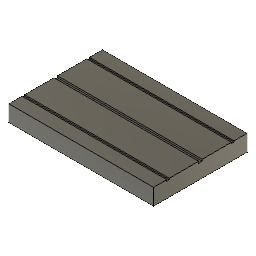
64 Halfsize Breadboard (Autodesk Fusion 360 design; units mm, degrees)
Autodesk Fusion 360 part; units mm, degrees
sketch "Sketch1" plane through (0, 0, 0) normal (0, 0, 1) x (1, 0, 0)
  line L0 (0, 0) -> (85, 0)
  line L1 (85, 0) -> (85, 55)
  line L2 (85, 55) -> (0, 55)
  line L3 (0, 55) -> (0, 0)
  dimension "d1" = 85
  dimension "d2" = 55
  measures "d1" distance of L0.start L0.end
  measures "d2" distance of L0.start L2.end
extrude "Extrude1" add sketch "Sketch1" along normal blind 9.7
sketch "Sketch2" plane through (0, 0, 9.7) normal (0, 0, 1) x (-1, 0, 0)
  line L0 (0, -55) -> (0, 0)
  line L1 (0, 0) -> (-85, 0)
  line L2 (-85, 0) -> (-85, -55)
  line L3 (-85, -55) -> (0, -55)
  line L4 (-85, -27.5) -> (0, -27.5)
  line L5 (0, -46.5) -> (-85, -46.5)
  line L6 (0, -8.5) -> (-85, -8.5)
  dimension "d5" = 19
  measures "d5" distance of L4 L5
pipe "Pipe1" cut square section size 2 path "Sketch2" along L4
pipe "Pipe2" cut square section size 1.5 path "Sketch2" along L6
pipe "Pipe3" cut square section size 1.5 path "Sketch2" along L5
